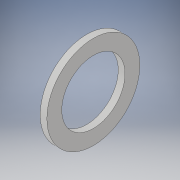
# Autodesk Inventor part: Pen Main Piece V3
Saved by Autodesk Inventor 2019 (Build 230136000, 136)
## iProperties
Created: 2019-06-10
Part Number: Pen Main Piece V3
Material: Generic
Document SubType Name: Modeling
Designer: Matthew XPS
Density: 1 g/cm^3
Appearance: Default
Author: Matthew XPS
Autodesk Inventor part; units mm, degrees
ref_plane "YZ Plane" through (0, 0, 0) normal (1, 0, 0) x (0, 1, 0)
ref_plane "XZ Plane" through (0, 0, 0) normal (0, 1, 0) x (-1, 0, 0)
ref_plane "XY Plane" through (0, 0, 0) normal (0, 0, 1) x (1, 0, 0)
sketch "Sketch2" plane through (0, 0, 0) normal (1, 0, 0) x (0, 1, 0)
  circle A0 centre (0, 0) radius 34.5
  circle A1 centre (0, 0) radius 23.5
  dimension "d4" = 69
  dimension "d5" = 11
  constraints: 2 centre point, 1 coincident
  measures "d4" diameter of A0
  measures "d5" radial gap between concentric circles of A0 A1
extrude "Extrusion1" add sketch "Sketch2" along normal blind 5
sketch "Sketch4" plane through (0, 0, 0) normal (1, 0, 0) x (0, 1, 0)
  line L0 (0, 0) -> (-13, 0)
  line L1 (-3.3346, -12.5651) -> (-13, 0)
  line L2 (-3.3346, -12.5651) -> (-3.3346, -24.054)
  line L3 (-3.3346, -12.5651) -> (-6.3346, -12.5651)
  line L4 (-13, 0) -> (-16, 0)
  line L5 (-13, 0) -> (-10, 0) construction
  line L6 (-16, 0) -> (-6.3346, -12.5651)
  line L7 (-6.3346, -12.5651) -> (-6.3346, -24.5651)
  line L8 (-3.3346, -24.054) -> (-6.3346, -24.5651)
  dimension "d16" = 13
  dimension "d17" = 13
  dimension "d18" = 52.431
  dimension "d20" = 3
  dimension "d21" = 3
  dimension "d22" = 180
  dimension "d50" = 12
  constraints: 18 end point, 3 horizontal, 2 vertical, 1 collinear, 1 perpendicular
  measures "d16" distance of L0.start L0.end
  measures "d17" distance of L0.start L1.start
  measures "d18" angle of L0 L1
  measures "d20" distance of L1.start L3.end
  measures "d21" distance of L0.end L4.end
  measures "d22" angle of L4 L5
  measures "d50" distance of L3.end L7.end
sketch "Sketch5" plane through (5, 0, 0) normal (1, 0, 0) x (0, 0, -1)
  circle A0 centre (0, 0) radius 23.5 projected
  circle A1 centre (0, 0) radius 34.5 projected
  arc A2 (-22.6301, -6.3346) -> (22.6301, -6.3346) centre (0, 0) ccw projected
  circle A3 centre (0, 0) radius 23.5
  line L0 (-24.5651, -6.3346) -> (-24.054, -3.3346) projected
  line L1 (-24.054, -3.3346) -> (-23.2622, -3.3346) projected
  arc A4 (23.2622, -3.3346) -> (-23.2622, -3.3346) centre (0, 0) ccw projected
  line L2 (23.2622, -3.3346) -> (24.054, -3.3346) projected
  line L3 (24.054, -3.3346) -> (24.5651, -6.3346) projected
  line L4 (-22.6301, -6.3346) -> (-24.5651, -6.3346) projected
  line L5 (24.5651, -6.3346) -> (22.6301, -6.3346) projected
  point P0 (20, 0)
  constraints: 1 centre point, 1 coincident, 1 concentric, 1 other
sketch "Sketch6" plane through (30, 0, 0) normal (-1, 0, 0) x (0, 0, 1)
  arc A0 (23.2622, -3.3346) -> (-23.2622, -3.3346) centre (0, 0) ccw projected
  circle A1 centre (0, 0) radius 34.5 projected
  arc A2 (-22.6301, -6.3346) -> (22.6301, -6.3346) centre (0, 0) ccw projected
  arc A3 (-23.2622, -3.3346) -> (-22.6301, -6.3346) centre (0, 0) ccw projected
  arc A4 (22.6301, -6.3346) -> (23.2622, -3.3346) centre (0, 0) ccw projected
sketch "Sketch9" plane through (30, 0, 0) normal (1, 0, 0) x (0, 0, -1)
  circle A0 centre (0, 0) radius 27.5
  circle A1 centre (0, -27.5) radius 3.1
  dimension "d32" = 55
  dimension "d33" = 6.2
  constraints: 1 centre point, 1 coincident, 1 vertical alignment, 2 other
  measures "d33" diameter of A1
sketch "Sketch10" plane through (30, 0, 0) normal (1, 0, 0) x (0, 0, -1)
  circle A0 centre (0, 0) radius 27.5
  circle A1 centre (27.5, 0) radius 3.5
  circle A2 centre (7.328, -26.5057) radius 2.5
  circle A3 centre (-7.328, -26.5057) radius 2.5
  circle A4 centre (-27.5, 0) radius 3.5
  circle A5 centre (0, 27.5) radius 3.5
  dimension "d39" = 55
  dimension "d40" = 7
  dimension "d41" = 5
  dimension "d42" = 5
  dimension "d43" = 7
  dimension "d44" = 7
  constraints: 6 centre point, 5 point on circle, 1 coincident
  measures "d39" diameter of A0
  measures "d40" diameter of A1
  measures "d41" diameter of A2
  measures "d42" diameter of A3
  measures "d43" diameter of A4
  measures "d44" diameter of A5
sketch "Sketch11" plane through (0, -6.3346, 12.5651) normal (0, -1, 0) x (1, 0, 0)
  line L0 (0, -35.8273) -> (0, 10.6972) projected
  line L1 (30, 0) -> (30, 10.0651) projected
  line L2 (30, 5.0325) -> (0, 5.0325)
  line L3 (0, 0) -> (0, 10.0651) projected
  circle A0 centre (15, 5.0325) radius 1.55
  line L4 (10, 5.0325) -> (10, 3.0325)
  line L5 (10, 5.0325) -> (12, 5.0325) construction
  circle A1 centre (10, 3.0325) radius 1.55
  line L6 (15, 5.0325) -> (15, 0.4582)
  circle A2 centre (20, 3.0325) radius 1.55
  point P0 (0, -12.5651)
  point P1 (20, 9.4891)
  point P2 (0, 9.4891)
  dimension "d47" = 3.1
  dimension "d51" = 2
  dimension "d52" = 90
  dimension "d53" = 3.1
  dimension "d64" = 5
  constraints: 8 end point, 3 centre point, 2 midpoint, 2 vertical, 1 coincident, 1 horizontal, 1 perpendicular, 1 point on line, 1 symmetric about line, 3 other
  measures "d47" diameter of A0
  measures "d51" distance of L4.start L4.end
  measures "d52" angle of L4 L5
  measures "d53" diameter of A1
  measures "d64" distance from line of L4.end L6
body "Solid1"
